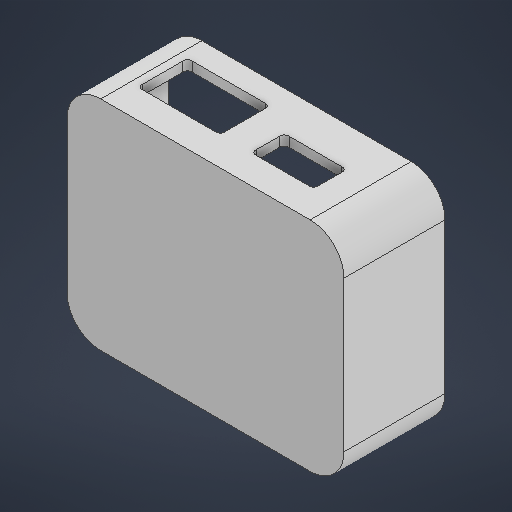
# Autodesk Inventor part: BottomShell
Saved by Autodesk Inventor 2026.2 (Build 302298000, 298)
## iProperties
Created: 2026-04-30
Part Number: BottomShell
Material: Generic
Document SubType Name: Modeling
Designer: FromDarkHell
Density: 1 g/cm^3
Appearance: Default
Author: FromDarkHell
Autodesk Inventor part; units mm, degrees
ref_plane "YZ Plane" through (0, 0, 0) normal (1, 0, 0) x (0, 1, 0)
ref_plane "XZ Plane" through (0, 0, 0) normal (0, 1, 0) x (-1, 0, 0)
ref_plane "XY Plane" through (0, 0, 0) normal (0, 0, 1) x (1, 0, 0)
sketch "Sketch1" plane through (0, 0, 0) normal (0, 0, 1) x (1, 0, 0)
  arc A0 (-152, -69.75) -> (-155, -72.75) centre (-152, -72.75) ccw projected
  line L0 (-155, -72.75) -> (-155, -103.75) projected
  line L1 (-155, -103.75) -> (-155, -104) projected
  arc A1 (-155, -104) -> (-152, -107) centre (-152, -104) ccw projected
  line L2 (-152, -107) -> (-108.5, -107) projected
  arc A2 (-108.5, -107) -> (-105.5, -104) centre (-108.5, -104) ccw projected
  line L3 (-105.5, -104) -> (-105.5, -103.75) projected
  line L4 (-105.5, -103.75) -> (-105.5, -72.75) projected
  arc A3 (-105.5, -72.75) -> (-108.5, -69.75) centre (-108.5, -72.75) ccw projected
  line L5 (-108.5, -69.75) -> (-152, -69.75) projected
  arc A4 (-111.5, -84.75) -> (-112.5, -83.75) centre (-112.5, -84.75) ccw projected
  line L6 (-111.5, -84.75) -> (-111.5, -99) projected
  arc A5 (-112.5, -100) -> (-111.5, -99) centre (-112.5, -99) ccw projected
  line L7 (-112.5, -100) -> (-114, -100) projected
  arc A6 (-115, -99) -> (-114, -100) centre (-114, -99) ccw projected
  line L8 (-115, -99) -> (-115, -90) projected
  arc A7 (-115, -90) -> (-116, -89) centre (-116, -90) ccw projected
  line L9 (-116, -89) -> (-120.0858, -89) projected
  arc A8 (-120.7929, -88.7071) -> (-120.0858, -89) centre (-120.0858, -87.9999) ccw projected
  line L10 (-120.7929, -88.7071) -> (-122.2071, -87.2929) projected
  arc A9 (-122.5, -86.5858) -> (-122.2071, -87.2929) centre (-121.5, -86.5858) ccw projected
  line L11 (-122.5, -86.5858) -> (-122.5, -84.75) projected
  arc A10 (-121.5, -83.75) -> (-122.5, -84.75) centre (-121.5, -84.75) ccw projected
  line L12 (-121.5, -83.75) -> (-112.5, -83.75) projected
  circle A11 centre (-137.75, -101) radius 0.5 projected
  circle A12 centre (-140.29, -101) radius 0.5 projected
  circle A13 centre (-142.83, -101) radius 0.5 projected
  circle A14 centre (-151, -102.75) radius 1.6 projected
  circle A15 centre (-137.69, -96.5) radius 0.5 projected
  circle A16 centre (-140.23, -96.5) radius 0.5 projected
  circle A17 centre (-142.77, -96.5) radius 0.5 projected
  circle A18 centre (-145.31, -96.5) radius 0.5 projected
  circle A19 centre (-109.75, -75) radius 1.6 projected
  circle A20 centre (-138.25, -79.11) radius 0.475 projected
  circle A21 centre (-140.75, -79.11) radius 0.475 projected
  circle A22 centre (-135.18, -76.4) radius 1.15 projected
  circle A23 centre (-142.75, -79.11) radius 0.475 projected
  circle A24 centre (-145.25, -79.11) radius 0.475 projected
  circle A25 centre (-148.32, -76.4) radius 1.15 projected
  arc A26 (-103.5, -72.75) -> (-108.5, -67.75) centre (-108.5, -72.75) ccw
  line L13 (-103.5, -72.75) -> (-103.5, -103.75)
  line L14 (-103.5, -103.75) -> (-103.5, -104)
  arc A27 (-108.5, -109) -> (-103.5, -104) centre (-108.5, -104) ccw
  line L15 (-108.5, -109) -> (-152, -109)
  arc A28 (-157, -104) -> (-152, -109) centre (-152, -104) ccw
  line L16 (-157, -104) -> (-157, -103.75)
  line L17 (-157, -103.75) -> (-157, -72.75)
  arc A29 (-152, -67.75) -> (-157, -72.75) centre (-152, -72.75) ccw
  line L18 (-152, -67.75) -> (-108.5, -67.75)
  line L19 (-152, -111) -> (-108.5, -111)
  arc A30 (-108.5, -111) -> (-101.5, -104) centre (-108.5, -104) ccw
  line L20 (-101.5, -104) -> (-101.5, -103.75)
  line L21 (-101.5, -103.75) -> (-101.5, -72.75)
  arc A31 (-101.5, -72.75) -> (-108.5, -65.75) centre (-108.5, -72.75) ccw
  line L22 (-108.5, -65.75) -> (-152, -65.75)
  arc A32 (-152, -65.75) -> (-159, -72.75) centre (-152, -72.75) ccw
  line L23 (-159, -72.75) -> (-159, -103.75)
  line L24 (-159, -103.75) -> (-159, -104)
  arc A33 (-159, -104) -> (-152, -111) centre (-152, -104) ccw
  point P0 (0, 0)
  dimension "d0" = 2
  dimension "d26" = 2
  constraints: 24 end point, 16 point on circle, 8 centre point, 18 other
  measures "d0" radial gap between concentric circles of A3 A26
  measures "d26" radial gap between concentric circles of A28 A33
extrude "Extrusion1" add sketch "Sketch1" along normal blind 2 contours L5 A3 L4 L3 A2 L2 A1 L1 L0 A0 | L6 A5 L7 A6 L8 A7 L9 A8 L10 A9 L11 A10 L12 A4 | A11 | A12 | A13 | A14 | A15 | A16 | A17 | A18 | A19 | A20 | A21 | A22 | A23 | A24 | A25 | L13 L14 A27 L15 A28 L16 L17 A29 L18 A26 | A33 L24 L23 A32 L22 A31 L21 L20 A30 L19
sketch "Sketch2" plane through (0, 0, 0) normal (0, 0, -1) x (-1, 0, 0)
  circle A0 centre (109.75, -75) radius 1.6 projected
  circle A1 centre (151, -102.75) radius 1.6 projected
  circle A2 centre (109.75, -75) radius 3.6
  circle A3 centre (151, -102.75) radius 3.6
  point P0 (0, 0)
  dimension "d3" = 2
  dimension "d4" = 2
  constraints: 2 centre point
  measures "d3" radial gap between concentric circles of A0 A2
  measures "d4" radial gap between concentric circles of A1 A3
extrude "Extrusion2" add sketch "Sketch2" along normal blind 4
sketch "Sketch3" plane through (0, 0, 0) normal (0, 0, -1) x (-1, 0, 0)
  arc A0 (155, -72.75) -> (152, -69.75) centre (152, -72.75) ccw projected
  line L0 (108.5, -69.75) -> (152, -69.75) projected
  arc A1 (108.5, -69.75) -> (105.5, -72.75) centre (108.5, -72.75) ccw projected
  line L1 (105.5, -103.75) -> (105.5, -72.75) projected
  line L2 (105.5, -104) -> (105.5, -103.75) projected
  arc A2 (105.5, -104) -> (108.5, -107) centre (108.5, -104) ccw projected
  line L3 (152, -107) -> (108.5, -107) projected
  arc A3 (152, -107) -> (155, -104) centre (152, -104) ccw projected
  line L4 (155, -103.75) -> (155, -104) projected
  line L5 (155, -72.75) -> (155, -103.75) projected
  arc A4 (112.5, -83.75) -> (111.5, -84.75) centre (112.5, -84.75) ccw projected
  line L6 (121.5, -83.75) -> (112.5, -83.75) projected
  arc A5 (122.5, -84.75) -> (121.5, -83.75) centre (121.5, -84.75) ccw projected
  line L7 (122.5, -86.5858) -> (122.5, -84.75) projected
  arc A6 (122.2071, -87.2929) -> (122.5, -86.5858) centre (121.5, -86.5858) ccw projected
  line L8 (120.7929, -88.7071) -> (122.2071, -87.2929) projected
  arc A7 (120.0858, -89) -> (120.7929, -88.7071) centre (120.0858, -87.9999) ccw projected
  line L9 (116, -89) -> (120.0858, -89) projected
  arc A8 (116, -89) -> (115, -90) centre (116, -90) ccw projected
  line L10 (115, -99) -> (115, -90) projected
  arc A9 (114, -100) -> (115, -99) centre (114, -99) ccw projected
  line L11 (112.5, -100) -> (114, -100) projected
  arc A10 (111.5, -99) -> (112.5, -100) centre (112.5, -99) ccw projected
  line L12 (111.5, -84.75) -> (111.5, -99) projected
  circle A11 centre (137.75, -101) radius 0.5 projected
  circle A12 centre (140.29, -101) radius 0.5 projected
  circle A13 centre (142.83, -101) radius 0.5 projected
  circle A14 centre (151, -102.75) radius 1.6 projected
  circle A15 centre (137.69, -96.5) radius 0.5 projected
  circle A16 centre (140.23, -96.5) radius 0.5 projected
  circle A17 centre (142.77, -96.5) radius 0.5 projected
  circle A18 centre (145.31, -96.5) radius 0.5 projected
  circle A19 centre (109.75, -75) radius 1.6 projected
  circle A20 centre (138.25, -79.11) radius 0.475 projected
  circle A21 centre (140.75, -79.11) radius 0.475 projected
  circle A22 centre (135.18, -76.4) radius 1.15 projected
  circle A23 centre (142.75, -79.11) radius 0.475 projected
  circle A24 centre (145.25, -79.11) radius 0.475 projected
  circle A25 centre (148.32, -76.4) radius 1.15 projected
  circle A26 centre (109.75, -75) radius 3.6 projected
  circle A27 centre (151, -102.75) radius 3.6 projected
  line L13 (157, -103.75) -> (157, -72.75) projected
  arc A28 (157, -72.75) -> (152, -67.75) centre (152, -72.75) ccw projected
  line L14 (152, -67.75) -> (108.5, -67.75) projected
  arc A29 (108.5, -67.75) -> (103.5, -72.75) centre (108.5, -72.75) ccw projected
  line L15 (103.5, -72.75) -> (103.5, -103.75) projected
  arc A30 (103.5, -104) -> (108.5, -109) centre (108.5, -104) ccw projected
  line L16 (108.5, -109) -> (152, -109) projected
  arc A31 (152, -109) -> (157, -104) centre (152, -104) ccw projected
  arc A32 (108.5, -65.75) -> (101.5, -72.75) centre (108.5, -72.75) ccw projected
  line L17 (108.5, -65.75) -> (152, -65.75) projected
  line L18 (101.5, -104) -> (101.5, -72.75) projected
  arc A33 (101.5, -104) -> (108.5, -111) centre (108.5, -104) ccw projected
  line L19 (152, -111) -> (108.5, -111) projected
  arc A34 (152, -111) -> (159, -104) centre (152, -104) ccw projected
  line L20 (159, -72.75) -> (159, -104) projected
  arc A35 (159, -72.75) -> (152, -65.75) centre (152, -72.75) ccw projected
  line L21 (103.5, -104) -> (103.5, -103.75)
  line L22 (157, -104) -> (157, -103.75)
  point P0 (0, 0)
  constraints: 4 end point, 1 parallel, 1 vertical
extrude "Extrusion3" add sketch "Sketch3" along normal blind 4 contours L17 A35 L20 A34 L19 A33 L18 A32
sketch "Sketch4" plane through (0, 0, -4) normal (0, 0, -1) x (-1, 0, 0)
  line L0 (155, -72.75) -> (155, -104) projected
  arc A0 (152, -107) -> (155, -104) centre (152, -104) ccw projected
  line L1 (152, -107) -> (108.5, -107) projected
  arc A1 (105.5, -104) -> (108.5, -107) centre (108.5, -104) ccw projected
  line L2 (105.5, -104) -> (105.5, -72.75) projected
  arc A2 (108.5, -69.75) -> (105.5, -72.75) centre (108.5, -72.75) ccw projected
  line L3 (108.5, -69.75) -> (152, -69.75) projected
  arc A3 (155, -72.75) -> (152, -69.75) centre (152, -72.75) ccw projected
  line L4 (148.3, -66.62) -> (148.3, -79.84) construction
  line L5 (135.2, -66.62) -> (135.2, -79.84) construction
  line L6 (124.72, -69.7975) -> (124.72, -76.6975) projected
  line L7 (115.78, -69.7975) -> (115.78, -76.6975) projected
  line L8 (136.55, -66.12) -> (146.95, -66.12) construction
  line L9 (124.72, -69.7975) -> (124.72, -67.75) construction
  line L10 (115.78, -69.7975) -> (115.78, -67.75) construction
  line L11 (150.3, -69.75) -> (150.3, -67.75)
  line L12 (133.2, -69.75) -> (133.2, -67.75)
  line L13 (126.72, -67.75) -> (126.72, -69.7975)
  line L14 (126.72, -69.7975) -> (126.72, -76.6975) construction
  line L15 (113.78, -67.75) -> (113.78, -69.7975)
  line L16 (113.78, -69.7975) -> (113.78, -76.6975) construction
  line L17 (101.5, -72.75) -> (101.5, -104) projected
  arc A4 (101.5, -104) -> (108.5, -111) centre (108.5, -104) ccw projected
  line L18 (108.5, -111) -> (152, -111) projected
  arc A5 (152, -111) -> (159, -104) centre (152, -104) ccw projected
  line L19 (159, -104) -> (159, -72.75) projected
  arc A6 (159, -72.75) -> (152, -65.75) centre (152, -72.75) ccw projected
  line L20 (152, -65.75) -> (108.5, -65.75) projected
  arc A7 (108.5, -65.75) -> (101.5, -72.75) centre (108.5, -72.75) ccw projected
  line L21 (155, -72.75) -> (155, -104) projected
  arc A8 (152, -107) -> (155, -104) centre (152, -104) ccw projected
  line L22 (152, -107) -> (108.5, -107) projected
  arc A9 (105.5, -104) -> (108.5, -107) centre (108.5, -104) ccw projected
  line L23 (105.5, -104) -> (105.5, -72.75) projected
  arc A10 (108.5, -69.75) -> (105.5, -72.75) centre (108.5, -72.75) ccw projected
  line L24 (108.5, -69.75) -> (152, -69.75) projected
  arc A11 (155, -72.75) -> (152, -69.75) centre (152, -72.75) ccw projected
  line L25 (150.3, -67.75) -> (150.3, -65.75)
  line L26 (133.2, -67.75) -> (133.2, -65.75)
  line L27 (126.72, -67.75) -> (126.72, -65.75)
  line L28 (113.78, -67.75) -> (113.78, -65.75)
  arc A12 (103.5, -104) -> (108.5, -109) centre (108.5, -104) ccw projected
  line L29 (152, -109) -> (108.5, -109) projected
  line L30 (103.5, -104) -> (103.5, -72.75) projected
  arc A13 (108.5, -67.75) -> (103.5, -72.75) centre (108.5, -72.75) ccw projected
  line L31 (108.5, -67.75) -> (152, -67.75) projected
  arc A14 (157, -72.75) -> (152, -67.75) centre (152, -72.75) ccw projected
  line L32 (152, -65.75) -> (108.5, -65.75) projected
  arc A15 (108.5, -65.75) -> (101.5, -72.75) centre (108.5, -72.75) ccw projected
  line L33 (101.5, -72.75) -> (101.5, -104) projected
  arc A16 (101.5, -104) -> (108.5, -111) centre (108.5, -104) ccw projected
  line L34 (108.5, -111) -> (152, -111) projected
  arc A17 (152, -111) -> (159, -104) centre (152, -104) ccw projected
  line L35 (159, -104) -> (159, -72.75) projected
  arc A18 (159, -72.75) -> (152, -65.75) centre (152, -72.75) ccw projected
  line L36 (103.5, -104) -> (103.5, -72.75) projected
  arc A19 (108.5, -67.75) -> (103.5, -72.75) centre (108.5, -72.75) ccw projected
  line L37 (108.5, -67.75) -> (152, -67.75) projected
  arc A20 (157, -72.75) -> (152, -67.75) centre (152, -72.75) ccw projected
  line L38 (157, -72.75) -> (157, -104) projected
  arc A21 (152, -109) -> (157, -104) centre (152, -104) ccw projected
  line L39 (152, -109) -> (108.5, -109) projected
  arc A22 (103.5, -104) -> (108.5, -109) centre (108.5, -104) ccw projected
  point P0 (0, 0)
  point P1 (126.72, -69.75)
  point P2 (113.78, -69.75)
  point P3 (157, -72.75)
  dimension "d9" = 2
  dimension "d10" = 2
  dimension "d11" = 2
  dimension "d12" = 2
  constraints: 24 end point, 6 point on line, 4 perpendicular, 2 other
  measures "d9" distance between parallel lines of L4 L11
  measures "d10" distance between parallel lines of L5 L12
  measures "d11" distance between parallel lines of L9 L13
  measures "d12" distance between parallel lines of L10 L15
extrude "Extrusion4" add sketch "Sketch4" along normal blind 15 contours L25 L20 A6 L19 A5 L18 A4 L17 A7 L28 L31 A13 L30 A12 L29 A21 L38 A14 | L31 L27 L20 L26
sketch "Sketch6" plane through (-152, -65.75, 2) normal (0, 1, 0) x (1, 0, 0)
  line L0 (15.45, 15.325) -> (5.05, 15.325) projected
  line L1 (31.75, 10.855) -> (28.53, 10.855) projected
  line L2 (31.75, 10.855) -> (34.97, 10.855) projected
  line L3 (15.45, 16.325) -> (5.05, 16.325)
  line L4 (5.05, 16.325) -> (2.7, 16.325)
  line L5 (15.45, 16.325) -> (17.8, 16.325)
  line L6 (1.7, 21) -> (18.8, 21)
  line L7 (1.7, 6) -> (1.7, 21) projected
  line L8 (18.8, 6) -> (18.8, 21) projected
  line L9 (25.28, 6) -> (25.28, 21) projected
  line L10 (38.22, 6) -> (38.22, 21) projected
  line L11 (1.7, 5.5) -> (1.7, 21) projected
  line L12 (1.7, 21) -> (1.7, 21)
  line L13 (18.8, 21) -> (18.8, 21)
  line L14 (17.8, 16.325) -> (18.8, 16.325)
  line L15 (2.7, 16.325) -> (1.7, 16.325)
  line L16 (28.53, 12.855) -> (31.75, 12.855)
  line L17 (31.75, 12.855) -> (34.97, 12.855)
  line L18 (28.53, 12.855) -> (25.28, 12.855)
  line L19 (34.97, 12.855) -> (38.22, 12.855)
  line L20 (25.28, 6) -> (38.22, 6) projected
  line L21 (1.7, 6) -> (18.8, 6) projected
  line L22 (0, 21) -> (43.5, 21) projected
  point P0 (152, 2)
  point P1 (18.8, 5.5)
  dimension "d15" = 1
  dimension "d27" = 2
  constraints: 24 end point, 7 point on line, 3 perpendicular, 2 equal length, 1 other
  measures "d15" distance between parallel lines of L0 L3
  measures "d27" distance between parallel lines of L1 L16
extrude "Extrusion5" add sketch "Sketch6" against normal blind 2 from surface at 0 contours L3 L4 L15 L7 L6 L8 L14 L5 | L9 L22 L10 L19 L17 L16 L18
fillet "Fillet1" radius 1 8 edges at (-126.72, -66.75, -4) (-113.78, -66.75, -4) (-133.2, -66.75, -14.325) (-133.2, -66.75, -4) (-150.3, -66.75, -4) (-150.3, -66.75, -14.325) (-113.78, -66.75, -10.855) (-126.72, -66.75, -10.855) curvature continuous yes
chamfer "Chamfer2" distance 2 angle 45 8 edges at (-130.25, -67.75, -19) (-155.5355, -69.2145, -19) (-157, -88.375, -19) (-155.5355, -107.5355, -19) (-130.25, -109, -19) (-104.9645, -107.5355, -19) (-103.5, -88.375, -19) (-104.9645, -69.2145, -19)
body "Solid1"
